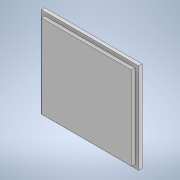
# Autodesk Inventor part: lid
Saved by Autodesk Inventor 2022 (Build 260153070, 153G)
## iProperties
Created: 2021-07-10
Part Number: lid
Material: 常规
Document SubType Name: Modeling
Designer: peter
Density: 1 g/cm^3
Appearance: 默认
Author: peter
Autodesk Inventor part; units mm, degrees
ref_plane "YZ Plane" through (0, 0, 0) normal (1, 0, 0) x (0, 1, 0)
ref_plane "XZ Plane" through (0, 0, 0) normal (0, 1, 0) x (-1, 0, 0)
ref_plane "XY Plane" through (0, 0, 0) normal (0, 0, 1) x (1, 0, 0)
sketch "草图5" plane through (0, 0, 0) normal (0, 0, 1) x (1, 0, 0)
  line L0 (0, 0) -> (140, 0)
  line L1 (140, 0) -> (140, 130)
  line L2 (140, 130) -> (0, 130)
  line L3 (0, 130) -> (0, 0)
  dimension "d10" = 140
  dimension "d11" = 130
  constraints: 8 end point, 2 parallel, 1 horizontal, 1 perpendicular
  measures "d10" distance of L2.end L1.end
  measures "d11" distance of L1.end L0.end
extrude "拉伸3" add sketch "草图5" along normal blind 5
sketch "草图6" plane through (0, 0, 5) normal (0, 0, 1) x (1, 0, 0)
  line L0 (5.1, 124.9) -> (134.9, 124.9)
  line L1 (134.9, 124.9) -> (134.9, 5.1)
  line L2 (134.9, 5.1) -> (5.1, 5.1)
  line L3 (5.1, 5.1) -> (5.1, 124.9)
  line L4 (140, 130) -> (0, 130) projected
  line L5 (0, 0) -> (140, 0) projected
  line L6 (0, 130) -> (0, 0) projected
  line L7 (140, 0) -> (140, 130) projected
  dimension "d14" = 129.8
  dimension "d15" = 119.8
  dimension "d22" = 5.1
  dimension "d23" = 5.1
  constraints: 8 end point, 2 parallel, 1 horizontal, 1 perpendicular
  measures "d14" distance of L1.end L2.end
  measures "d15" distance of L0.end L1.end
  measures "d22" distance between parallel lines of L7 L1
  measures "d23" distance between parallel lines of L5 L2
extrude "拉伸4" add sketch "草图6" along normal blind 5 contours L0 L1 L2 L3
